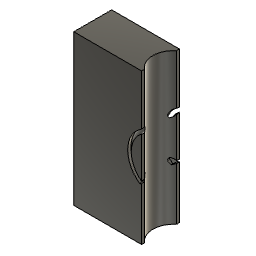
case (Autodesk Fusion 360 design; units mm, degrees)
Autodesk Fusion 360 part; units mm, degrees
note: some values were not read from the file. Set by a fixed rule: which sketch regions a step uses.
sketch "Sketch2" plane through (0, 0, 0) normal (0, 0, 1) x (1, 0, 0)
  line L0 (0, 0) -> (53.6, 0)
  arc A0 (67.2, 0) -> (40, 0) centre (53.6, 0) ccw
  line L1 (53.6, 0) -> (67.2, 0)
  line L2 (0, 0) -> (0, 12.6)
  line L3 (0, 12.6) -> (48.4814, 12.6)
  line L4 (45.0794, 12.6) -> (45.0794, 10.6)
  dimension "d11" = 27.2
  dimension "d18" = 40
  dimension "d19" = 12.6
  dimension "d20" = 2
  constraint coincident L0.start L2.start
  constraint horizontal L0
  constraint coincident L0 A0.end
  constraint coincident L0.end A0.centre
  constraint parallel L0 L1
  constraint perpendicular L0 L2
  constraint coincident A0 L3.end
  constraint perpendicular L2 L3
  constraint coincident L3 L4.start
  constraint coincident A0 L4.end
  constraint perpendicular L3 L4
  measures "d11" distance of A0.start A0.end
  measures "d18" distance of L0.start A0.end
  measures "d19" distance of L0.start L2.end
  measures "d20" distance of L4.start L4.end
extrude "Extrude4" add sketch "Sketch2" along normal mid plane 100 contours L0 A0 L2 L3 L4 makes body 1
mirror "Mirror2" about plane through (0, 0, 0) normal (0, 1, 0) of "Extrude4" makes body 2
combine "Combine1" operation add target body 2 tool bodies 1
sketch "Sketch3" plane through (0, 0, 0) normal (-1, 0, 0) x (0, -1, 0)
  line L0 (-12.6, -50) -> (12.6, -50)
  line L1 (12.6, -50) -> (12.6, 50)
  line L2 (12.6, 50) -> (-12.6, 50)
  line L3 (-12.6, 50) -> (-12.6, -50)
  line L4 (-10.6, 48) -> (10.6, 48)
  line L5 (10.6, 48) -> (10.6, 40.2)
  line L6 (10.6, 40.2) -> (-10.6, 40.2)
  line L7 (-10.6, 40.2) -> (-10.6, 48)
  dimension "d26" = 2
  dimension "d27" = 2
  dimension "d28" = 2
  dimension "d32" = 7.8
  constraint horizontal L4
  constraint vertical L5
  constraint horizontal L6
  constraint vertical L7
  measures "d26" horizontal distance of L1.end L4.end
  measures "d27" vertical distance of L1.end L4.end
  measures "d28" horizontal distance of L2.end L4.start
  measures "d32" distance of L4.end L5.end
extrude "Extrude5" cut sketch "Sketch3" against normal blind 1.5 contours L4 L5 L6 L7 bodies 2
fillet "Fillet1" radius 2 4 edges at (0.75, 10.6, 48) (0.75, 10.6, 40.2) (0.75, -10.6, 48) (0.75, -10.6, 40.2) on bodies 2
pattern_linear "R-Pattern2" count 10 spacing 9.8 along (0, 0, -1) of "Extrude5", "Fillet1"
sketch "Sketch5" plane through (0, -12.6, 0) normal (0, -1, 0) x (1, 0, 0)
  line L0 (0, 50) -> (0, -50) construction
  line L1 (0, -50) -> (45.0794, -50) construction
  line L2 (45.0794, -50) -> (45.0794, 50)
  line L3 (45.0794, 50) -> (0, 50) construction
  arc A0 (45.0794, 15) -> (45.0794, -15) centre (55.1419, 0) ccw
  line L4 (45.0794, 0) -> (55.1419, 0) construction
  line L5 (45.0794, 0) -> (37.0794, 0) construction
  dimension "d89" = 30
  dimension "d90" = 8
  constraint coincident L2 A0.start
  constraint coincident L2 A0.end
  constraint midpoint L2 L4.start
  constraint perpendicular L2 L4
  constraint coincident A0.centre L4.end
  constraint midpoint A0 L5.end
  measures "d89" distance of A0.end A0.start
  measures "d90" distance of L4.start L5.end
ref_plane "WorkPlane1" through (45.0794, 0, 0) normal (1, 0, 0) x (0, 1, 0)
sketch "Sketch6" plane through (45.0794, 0, 0) normal (1, 0, 0) x (0, 1, 0)
  circle A0 centre (-9.6, 15) radius 2
  line L0 (-10.0209, 16.9552) -> (-12.6, 16.4)
  line L1 (-12.6, 15) -> (-12.6, 16.4)
  line L2 (-9.6, 15) -> (-12.6, 15) construction
  line L3 (-10.0209, 13.0448) -> (-12.6, 13.6)
  line L4 (-12.6, 13.6) -> (-12.6, 15)
  point P0 (-12.6, 15)
  dimension "d53" = 4
  dimension "d54" = 1.4
  dimension "d58" = 3
  constraint coincident A0 L0.start
  constraint vertical L1
  constraint tangent A0 L0
  constraint coincident A0.centre L2.start
  constraint horizontal L2
  constraint symmetric L0.start L2 L3.start
  constraint symmetric L0.end L2 L3.end
  constraint coincident P0 L1.start
  measures "d53" diameter of A0
  measures "d54" distance of L0.end P0
  measures "d58" distance of A0.centre P0
sweep "Sweep1" cut profiles "Sketch6" path "Sketch5" along A0 section 1 bodies 2
mirror "Mirror3" about plane through (0, 0, 0) normal (0, 1, 0) of "Sweep1"
sketch "Sketch9" plane through (0, 0, 0) normal (0, 0, 1) x (1, 0, 0)
  line L0 (3, 9.6) -> (37, 9.6)
  line L1 (37, 9.6) -> (37, -9.6)
  line L2 (3, -9.6) -> (3, 9.6)
  line L3 (3, 0) -> (37, 0) construction
  line L4 (3, -9.6) -> (37, -9.6)
  line L5 (3, 0) -> (0, 0) construction
  circle A0 centre (27.5, 0) radius 11
  line L6 (40, 0) -> (37, 0) construction
  point P0 (0, 12.6)
  point P1 (40, 0)
  point P2 (38.5, 0)
  dimension "d73" = 3
  dimension "d76" = 3
  dimension "d77" = 3
  dimension "d78" = 22
  dimension "d81" = 1.5
  constraint horizontal L0
  constraint vertical L1
  constraint vertical L2
  constraint coincident L2 L3.start
  constraint coincident L1 L3.end
  constraint perpendicular L1 L3
  constraint symmetric L0.start L3 L2.start
  constraint symmetric L0.end L3 L1.end
  constraint coincident L5.end origin
  constraint horizontal L5
  constraint coincident L3 A0.centre
  constraint coincident A0 P2
  constraint coincident P1 L6.start
  constraint coincident P2 L6
  measures "d73" horizontal distance of P0 L0.start
  measures "d76" distance of L1 P1
  measures "d77" vertical distance of P0 L0.start
  measures "d78" diameter of A0
  measures "d81" distance of P2 P1
extrude "Extrude7" cut sketch "Sketch9" along normal mid plane 94 contours L0 L2 L4 A0 | L0 A0 | L0 L1 L4 A0 | L4 A0 | L1 A0 bodies 2
sketch "Sketch10" plane through (0, 0, -50) normal (0, 0, -1) x (1, 0, 0)
  arc A0 (45.0794, 10.6) -> (45.0794, -10.6) centre (53.6, 0) ccw
  line L0 (45.0794, 10.6) -> (45.0794, 12.6)
  line L1 (45.0794, 12.6) -> (0, 12.6)
  line L2 (0, 12.6) -> (0, -12.6)
  line L3 (0, -12.6) -> (45.0794, -12.6)
  line L4 (45.0794, -12.6) -> (45.0794, -10.6)
  arc A1 (43.3628, 11.1) -> (43.3628, -11.1) centre (53.6, 0) ccw
  line L5 (1.5, -11.1) -> (43.3628, -11.1)
  line L6 (1.5, 11.1) -> (1.5, -11.1)
  line L7 (43.3628, 11.1) -> (1.5, 11.1)
  dimension "d83" = -1.5
extrude "Extrude8" cut sketch "Sketch10" against normal blind 3 contours A1 L5 L6 L7 bodies 2
extrude "Extrude9" add sketch "Sketch10" against normal blind 3 separate body contours A1 L5 L6 L7 makes body 3
sketch "Sketch11" plane through (0, 0, -47) normal (0, 0, -1) x (1, 0, 0)
  line L0 (43.3628, 11.1) -> (1.5, 11.1)
  line L1 (1.5, 11.1) -> (1.5, 10.3321)
  line L2 (1.5, -11.1) -> (43.3628, -11.1)
  arc A0 (38.5, 0) -> (43.3628, -11.1) centre (53.6, 0) ccw
  arc A1 (22.1297, -9.6) -> (38.5, 0) centre (27.5, 0) ccw
  line L3 (22.1297, -9.6) -> (3, -9.6)
  line L4 (3, -9.6) -> (3, 9.6)
  line L5 (3, 9.6) -> (22.1297, 9.6)
  arc A2 (38.5, 0) -> (22.1297, 9.6) centre (27.5, 0) ccw
  arc A3 (43.3628, 11.1) -> (38.5, 0) centre (53.6, 0) ccw
  line L6 (3, -9.6) -> (3, -11.1)
  line L7 (3, 9.6) -> (3, 11.1)
  line L8 (1.5, 10.3321) -> (1.5, -10.3321)
  line L9 (1.5, -10.3321) -> (1.5, -11.1)
  constraint coincident L2 L6.end
  constraint perpendicular L2 L6
  constraint coincident L0 L7.end
  constraint perpendicular L0 L7
  constraint coincident L4.end L5.start
  constraint coincident L3.end L4.start
extrude "Extrude10" cut sketch "Sketch11" against normal blind 94 contours L0 L1 L2 L4 L6 L7 L8 L9 bodies 2
sketch "Sketch12" plane through (0, -9.6, 0) normal (0, 1, 0) x (-1, 0, 0)
  line L0 (-22.1297, 47) -> (-22.1297, -47)
  line L1 (-22.1297, -47) -> (-3, -47)
  line L2 (-3, -47) -> (-3, 47)
  line L3 (-3, 47) -> (-22.1297, 47)
extrude "Extrude11" add sketch "Sketch11" against normal up to surface (94 mm away) separate body contours L0 L1 L2 L4 L6 L7 L8 L9 makes body 4
hidden bodies 4
equation "seatpost_dia = 27.2 mm"
equation "backside_min = 2 mm"
equation "d11 = seatpost_dia"
equation "depth = 40 mm"
equation "seatpost_overlap = -2 mm"
equation "d18 = depth"
equation "d19 = ( seatpost_dia + seatpost_overlap ) / 2"
equation "d20 = backside_min"
equation "d21 = height"
equation "led_line_offset = 2 mm"
equation "d26 = led_line_offset"
equation "d27 = led_line_offset"
equation "d28 = led_line_offset"
equation "led_lien_count = 10"
equation "height = 100 mm"
equation "d32 = ( height - ( led_line_offset * ( led_lien_count + 1 ) ) ) / led_lien_count"
equation "d33 = -shell_thickness / 2"
equation "led_line_height = ( height - ( led_line_offset * ( led_lien_count + 1 ) ) ) / led_lien_count"
equation "d41 = light_rounding"
equation "light_rounding = 2 mm"
equation "d44 = led_lien_count"
equation "d46 = led_line_height + led_line_offset"
equation "rubber_band_hole_size = 4 mm"
equation "rubber_band_circle_height = 30 mm"
equation "d53 = rubber_band_hole_size"
equation "d54 = ( rubber_band_hole_size / 2 ) * 0.70"
equation "d58 = rubber_band_hole_size * 0.75"
equation "shell_thickness = 3 mm"
equation "d73 = shell_thickness"
equation "d76 = shell_thickness"
equation "d77 = shell_thickness"
equation "d82 = height - shell_thickness * 2"
equation "d83 = -shell_thickness / 2"
equation "d84 = -shell_thickness"
equation "d86 = -shell_thickness"
equation "rubber_band_circle_depth = 8 mm"
equation "d89 = rubber_band_circle_height"
equation "d90 = rubber_band_circle_depth"
